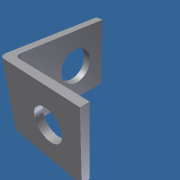
# Autodesk Inventor part: LCouplerSmall
Saved by Autodesk Inventor 2012 (Build 160160000, 160)
## iProperties
Created: 2014-01-28
Part Number: LCouplerSmall
Material: Default
Document SubType Name: Modeling
Designer: Admin
Density: 1 g/cm^3
Author: Admin
Autodesk Inventor part; units mm, degrees
ref_plane "YZ Plane" through (0, 0, 0) normal (1, 0, 0) x (0, 1, 0)
ref_plane "XZ Plane" through (0, 0, 0) normal (0, 1, 0) x (-1, 0, 0)
ref_plane "XY Plane" through (0, 0, 0) normal (0, 0, 1) x (1, 0, 0)
sketch "Sketch1" plane through (0, 0, 0) normal (0, 0, 1) x (1, 0, 0)
  line L0 (0, -2.2666) -> (0, 12.7444) projected
  line L1 (0, 10.6) -> (0, 0.59)
  line L2 (8.9, 0) -> (8.9, 0.82)
  line L3 (8.9, 0.82) -> (1.41, 0.82)
  line L4 (0.82, 1.41) -> (0.82, 10.6)
  line L5 (0, 10.6) -> (0.82, 10.6)
  line L6 (0.59, 0) -> (8.9, 0)
  arc A0 (0.82, 1.41) -> (1.41, 0.82) centre (1.41, 1.41) ccw
  arc A1 (0, 0.59) -> (0.59, 0) centre (0.59, 0.59) ccw
  point P0 (0, 0)
  dimension "d0" = 10.6
  dimension "d1" = 8.9
  dimension "d2" = 0.82
  dimension "d3" = 0.82
  dimension "d4" = 0.59
  constraints: 12 end point, 4 point on circle, 4 tangent, 3 parallel, 3 point on line, 2 centre point, 2 perpendicular, 1 equal radius
  measures "d0" distance of L1.start point (0, 0)
  measures "d1" distance of point (0, 0) L2.start
  measures "d2" distance between parallel lines of L6 L3
  measures "d3" distance between parallel lines of L0 L4
  measures "d4" radius of A0
extrude "Extrusion1" add sketch "Sketch1" along normal blind 7.2
sketch "Sketch2" plane through (1.41, 0.82, 0) normal (0, 1, 0) x (1, 0, 0)
  line L0 (0, -7.2) -> (7.49, -7.2) projected
  circle A0 centre (3.99, -3.6) radius 1.6
  line L1 (7.49, 0) -> (7.49, -7.2) projected
  point P0 (-1.41, 0)
  dimension "d7" = 3.5
  dimension "d8" = 3.2
  dimension "d9" = 3.6
  constraints: 1 centre point
  measures "d7" distance from line of L1 A0.centre
  measures "d8" diameter of A0
  measures "d9" distance from line of L0 A0.centre
extrude "Extrusion2" cut sketch "Sketch2" against normal through all
sketch "Sketch3" plane through (0.82, 1.41, 0) normal (1, 0, 0) x (0, 0, -1)
  line L0 (0, 0) -> (0, 9.19) projected
  line L1 (0, 9.19) -> (-7.2, 9.19) projected
  circle A0 centre (-3.6, 5.69) radius 1.825
  point P0 (0, -1.41)
  dimension "d12" = 3.65
  dimension "d13" = 3.5
  dimension "d14" = 3.6
  constraints: 1 centre point
  measures "d12" diameter of A0
  measures "d13" distance from line of A0.centre L1
  measures "d14" distance from line of L0 A0.centre
extrude "Extrusion3" cut sketch "Sketch3" against normal through all
body "Solid1"
